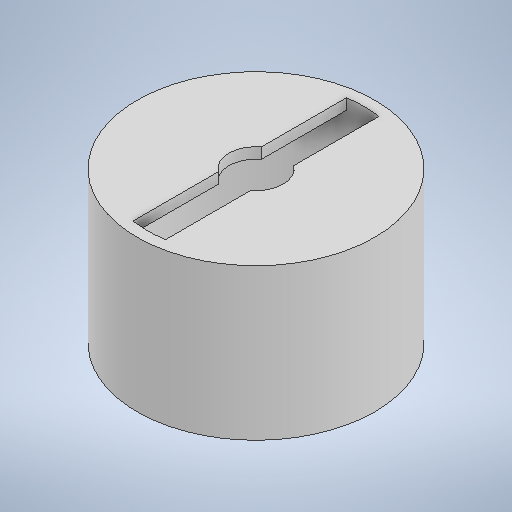
# Autodesk Inventor part: LED-Schirm
Saved by Autodesk Inventor 2025.1 (Build 291241000, 241)
## iProperties
Created: 2025-01-26
Part Number: LED-Schirm
Material: Generisch
Document SubType Name: Modeling
Designer: joebe
Density: 1 g/cm^3
Appearance: Vorgabe
Author: joebe
Autodesk Inventor part; units mm, degrees
ref_plane "YZ Plane" through (0, 0, 0) normal (1, 0, 0) x (0, 1, 0)
ref_plane "XZ Plane" through (0, 0, 0) normal (0, 1, 0) x (-1, 0, 0)
ref_plane "XY Plane" through (0, 0, 0) normal (0, 0, 1) x (1, 0, 0)
sketch "Skizze1" plane through (0, 0, 0) normal (0, 0, 1) x (1, 0, 0)
  circle A0 centre (0, 0) radius 11
  dimension "d0" = 22
  constraints: 1 centre point, 1 coincident
  measures "d0" diameter of A0
extrude "Extrusion1" add sketch "Skizze1" along normal mid plane 14
sketch "Skizze2" plane through (0, 0, -7) normal (0, 0, -1) x (-1, 0, 0)
  circle A0 centre (0, 0) radius 10
  circle A1 centre (0, 0) radius 11 projected
  dimension "d3" = 1
  constraints: 1 centre point, 1 coincident
  measures "d3" radial gap between concentric circles of A1 A0
extrude "Extrusion2" cut sketch "Skizze2" against normal blind 13 contours A0
sketch "Skizze3" plane through (0, 0, 7) normal (0, 0, 1) x (1, 0, 0)
  circle A0 centre (0, 0) radius 2.5
  circle A1 centre (0, 0) radius 10 projected
  line L0 (1.5, -9.8869) -> (1.5, 9.8869)
  line L1 (-1.5, -9.8869) -> (-1.5, 9.8869)
  point P0 (-1.5, 2)
  point P1 (-1.5, -2)
  point P2 (1.5, -2)
  point P3 (1.5, 2)
  dimension "d6" = 5
  dimension "d7" = 3
  dimension "d8" = 1.5
  constraints: 4 end point, 4 point on circle, 1 centre point, 1 coincident, 1 parallel, 1 vertical
  measures "d6" diameter of A0
  measures "d7" distance between parallel lines of L0 L1
  measures "d8" distance from line of point (0, 0) L0
extrude "Extrusion3" cut sketch "Skizze3" against normal blind 11 contours A0 L0 | L0 A0 L1 | A0 L1 A1 L0 | L0 A1 L1 A0 | L1 A0
equation "\"d8\" = 0.5 * d7"
